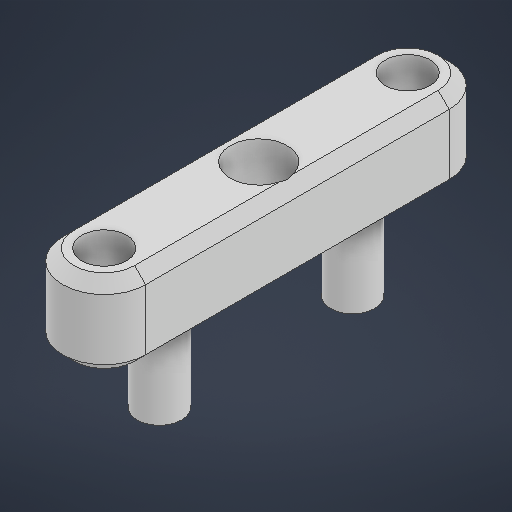
# Autodesk Inventor part: Gear_Holder_1
Saved by Autodesk Inventor 2026.2 (Build 302298000, 298)
## iProperties
Created: 2025-12-19
Part Number: Gear_Holder_1
Material: Generic
Document SubType Name: Modeling
Designer: Cobble
Density: 1 g/cm^3
Appearance: Default
Author: Cobble
Autodesk Inventor part; units mm, degrees
ref_plane "YZ Plane" through (0, 0, 0) normal (1, 0, 0) x (0, 1, 0)
ref_plane "XZ Plane" through (0, 0, 0) normal (0, 1, 0) x (-1, 0, 0)
ref_plane "XY Plane" through (0, 0, 0) normal (0, 0, 1) x (1, 0, 0)
sketch "Sketch1" plane through (0, 0, 0) normal (0, 0, 1) x (1, 0, 0)
  line L0 (0, 0) -> (15, 0)
  line L1 (15, 0) -> (15, 70)
  line L2 (15, 70) -> (0, 70)
  line L3 (0, 70) -> (0, 0)
  line L4 (15, 35) -> (0, 35)
  line L5 (0, 60) -> (15, 60)
  line L6 (15, 60) -> (15, 10)
  line L7 (15, 10) -> (0, 10)
  line L8 (0, 10) -> (0, 60)
  line L9 (0, 60) -> (15, 10) construction
  line L10 (15, 60) -> (0, 10) construction
  line L11 (7.5, 35) -> (8, 35)
  circle A0 centre (8, 35) radius 5.15
  line L12 (0, 0) -> (15, 0)
  line L13 (15, 0) -> (15, 15)
  line L14 (15, 15) -> (0, 15) construction
  line L15 (0, 15) -> (0, 0)
  line L16 (0, 70) -> (15, 70)
  line L17 (15, 70) -> (15, 55)
  line L18 (15, 55) -> (0, 55) construction
  line L19 (0, 55) -> (0, 70)
  line L20 (15, 15) -> (0, 0) construction
  line L21 (0, 70) -> (15, 55) construction
  circle A1 centre (7.5, 7.5) radius 7.5
  circle A2 centre (7.5, 62.5) radius 7.5
  line L22 (0, 10) -> (15, 10)
  line L23 (15, 10) -> (15, 25)
  line L24 (15, 25) -> (0, 25)
  line L25 (0, 25) -> (0, 10)
  line L26 (15, 60) -> (0, 60)
  line L27 (0, 60) -> (0, 45)
  line L28 (0, 45) -> (15, 45)
  line L29 (15, 45) -> (15, 60)
  line L30 (0, 45) -> (15, 60) construction
  line L31 (0, 10) -> (15, 25) construction
  circle A3 centre (7.5, 17.5) radius 4
  circle A4 centre (7.5, 52.5) radius 4
  circle A5 centre (7.5, 7.5) radius 4.05
  circle A6 centre (7.5, 62.5) radius 4.05
  point P0 (15, 7.5)
  point P1 (15, 62.5)
  point P2 (0, 62.5)
  point P3 (0, 7.5)
  point P4 (7.5, 70)
  point P5 (7.5, 0)
  dimension "d0" = 15
  dimension "d1" = 70
  dimension "d2" = 15
  dimension "d3" = 50
  dimension "d5" = 0.5
  dimension "d6" = 10.3
  dimension "d7" = 15
  dimension "d8" = 15
  dimension "d9" = 15
  dimension "d10" = 15
  dimension "d11" = 15
  dimension "d12" = 15
  dimension "d13" = 15
  dimension "d14" = 15
  dimension "d15" = 8
  dimension "d16" = 8
  dimension "d26" = 8.1
  dimension "d27" = 8.1
  constraints: 64 end point, 12 parallel, 7 centre point, 7 midpoint, 6 horizontal, 6 perpendicular, 3 coincident, 2 tangent, 1 point on line
  measures "d0" distance of L2.end L1.end
  measures "d1" distance of L1.end L0.end
  measures "d2" distance of L6.end L7.end
  measures "d3" distance of L5.end L6.end
  measures "d5" distance of L11.start L11.end
  measures "d6" diameter of A0
  measures "d7" distance of L14.end L13.end
  measures "d8" distance of L13.end L12.end
  measures "d9" distance of L17.end L18.end
  measures "d10" distance of L16.end L17.end
  measures "d11" distance of L24.end L23.end
  measures "d12" distance of L23.end L22.end
  measures "d13" distance of L28.end L27.end
  measures "d14" distance of L27.end L26.end
  measures "d15" diameter of A3
  measures "d16" diameter of A4
  measures "d26" diameter of A5
  measures "d27" diameter of A6
extrude "Extrusion1" add sketch "Sketch1" against normal blind 15 contours A3 A1 | A1 A3 | A4 A2 | A2 A4
extrude "Extrusion2" add sketch "Sketch1" along normal blind 15 contours L3 A1 L0 | A1 L1 L0 | A1 L7 A5 | L3 L7 A1 | A1 L7 L1 | L3 L24 L1 L7 A1 A3 | A1 A3 L7 A5 | A3 A1 | A1 A3 | L3 L4 A0 L1 L24 | L3 L28 L1 L4 A0 | L3 L5 A2 A4 L1 L28 | L3 A2 L5 | L5 A2 L1 | L3 L2 A2 | A2 L5 A6 | L5 A6 A2 A4 | A2 L2 L1 | A4 A2 | A2 A4
fillet "Fillet2" radius 7.5 4 edges at (15, 0, 7.5) (0, 0, 7.5) (15, 70, 7.5) (0, 70, 7.5)
chamfer "Chamfer2" distance 2 angle 45 12 edges at (12.8033, 67.8033, 15) (12.8033, 2.1967, 15) (2.1967, 67.8033, 15) (2.1967, 2.1967, 15) (0, 35, 15) (15, 35, 15) (15, 35, 0) (12.8033, 67.8033, 0) (12.8033, 2.1967, 0) (2.1967, 67.8033, 0) (2.1967, 2.1967, 0) (0, 35, 0)
body "Solid1"
